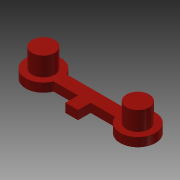
# Autodesk Inventor part: fwd_rev_btns
Saved by Autodesk Inventor 2014 (Build 180170000, 170)
## iProperties
Created: 2017-11-19
Part Number: fwd_rev_btns
Material: Типовые
Document SubType Name: Modeling
Designer: Nikopol
Density: 1 g/cm^3
Appearance: Оранжево-красный
Author: Nikopol
Autodesk Inventor part; units mm, degrees
ref_plane "YZ Plane" through (0, 0, 0) normal (1, 0, 0) x (0, 1, 0)
ref_plane "XZ Plane" through (0, 0, 0) normal (0, 1, 0) x (-1, 0, 0)
ref_plane "XY Plane" through (0, 0, 0) normal (0, 0, 1) x (1, 0, 0)
sketch "Эскиз1" plane through (0, 0, 0) normal (0, 0, 1) x (1, 0, 0)
  arc A0 (-4.8847, 1) -> (-4.8847, -1) centre (-7.5, 0) ccw
  arc A1 (4.8847, -1) -> (4.8847, 1) centre (7.5, 0) ccw
  line L0 (-7.5, 0) -> (7.5, 0) construction
  line L1 (-4.8847, 1) -> (4.8847, 1)
  line L2 (1, -1) -> (1, -3)
  line L3 (1, -3) -> (-1, -3)
  line L4 (-1, -3) -> (-1, -1)
  line L5 (-4.8847, -1) -> (-1, -1)
  line L6 (1, -1) -> (4.8847, -1)
  point P0 (0, 0)
  point P1 (0, 1)
  point P2 (0, -3)
  point P3 (0, 0)
  dimension "d0" = 5.6
  dimension "d1" = 5.6
  dimension "d2" = 15
  dimension "d3" = 1
  dimension "d7" = 2
  dimension "d8" = 2
  constraints: 14 end point, 4 parallel, 4 point on circle, 3 midpoint, 2 centre point, 2 vertical alignment, 1 horizontal
  measures "d0" diameter of A0
  measures "d1" diameter of A1
  measures "d2" distance of L0.end L0.start
  measures "d3" distance between parallel lines of L0 L1
  measures "d7" distance of L3.end L4.end
  measures "d8" distance of L2.end L3.end
extrude "Выдавливание1" add sketch "Эскиз1" along normal blind 1.4
sketch "Эскиз2" plane through (0, 0, 1.4) normal (0, 0, 1) x (1, 0, 0)
  arc A0 (-4.8847, 1) -> (-4.8847, -1) centre (-7.5, 0) ccw projected
  arc A1 (4.8847, -1) -> (4.8847, 1) centre (7.5, 0) ccw projected
  circle A2 centre (-7.5, 0) radius 1.8
  circle A3 centre (7.5, 0) radius 1.8
  point P0 (0, 0)
  dimension "d11" = 3.6
  dimension "d12" = 3.6
  constraints: 2 centre point, 2 coincident
  measures "d11" diameter of A2
  measures "d12" diameter of A3
extrude "Выдавливание2" add sketch "Эскиз2" along normal blind 3
